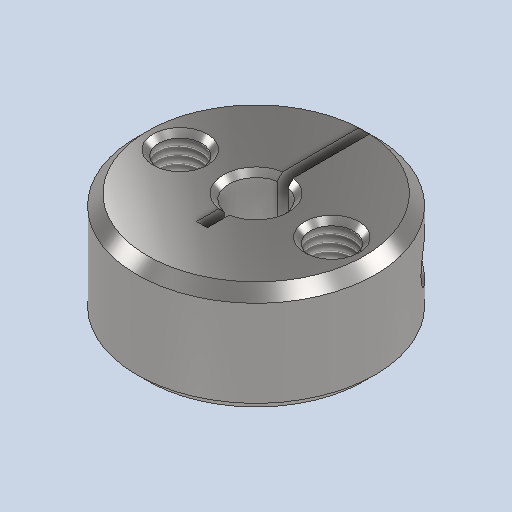
# Autodesk Inventor part: setcorer_5-10-22
Saved by Autodesk Inventor 2025.1 (Build 291241000, 241)
## iProperties
Created: 2023-12-06
Part Number: setcorer_5-10-22
Material: ステンレス鋼 440C
Document SubType Name: Modeling
Designer: fhbdh
Density: 7.75 g/cm^3
Appearance: 半つや出し
Author: fhbdh
Autodesk Inventor part; units mm, degrees
ref_plane "XZ Plane" through (0, 0, 0) normal (0, 1, 0) x (-1, 0, 0)
ref_plane "XY Plane" through (0, 0, 0) normal (0, 0, 1) x (1, 0, 0)
sketch "スケッチ1" plane through (0, 0, 0) normal (0, 1, 0) x (-1, 0, 0)
  circle A0 centre (0, 0) radius 11
  circle A1 centre (0, 0) radius 2.5
  line L0 (0.5, 5) -> (0.5, -10.9886)
  line L1 (0.5, 5) -> (-0.5, 5)
  line L2 (-0.5, 5) -> (-0.5, -10.9886)
  line L3 (0, 0) -> (0, -11) construction
  circle A2 centre (7, 0) radius 2
  line L4 (0, 0) -> (7, 0) construction
  circle A3 centre (-7, 0) radius 2
  point P0 (0.5, 2.4495)
  point P1 (0.5, -2.4495)
  point P2 (-0.5, -2.4495)
  point P3 (-0.5, 2.4495)
  dimension "d0" = 22
  dimension "d1" = 5
  dimension "d2" = 1
  dimension "d3" = 16
  dimension "d4" = 4
  dimension "d7" = 360
  dimension "d9" = 14
  constraints: 10 end point, 4 centre point, 3 point on circle, 2 coincident, 2 horizontal, 2 vertical, 1 parallel, 6 other
  measures "d0" diameter of A0
  measures "d1" diameter of A1
  measures "d2" distance between parallel lines of L2 L0
  measures "d3" distance from line of L3.end L1
  measures "d4" diameter of A2
  measures "d9" distance of A3.centre L4.end
extrude "押し出し1" add sketch "スケッチ1" along normal blind 10 contours A0 L0 A1 L1 L2
ref_plane "作業平面1" through (-11, 0, 0) normal (1, 0, 0) x (0, 1, 0)
sketch "スケッチ2" plane through (-11, 0, 0) normal (1, 0, 0) x (0, 1, 0)
  line L0 (0, 11) -> (10, 11) projected
  line L1 (5, 11) -> (5, -10.9886) construction
  line L2 (0, -10.9886) -> (10, -10.9886) projected
  circle A0 centre (5, -8) radius 4
  point P0 (0, 0)
  dimension "d12" = 8
  dimension "d13" = 8
  constraints: 2 end point, 2 midpoint, 1 centre point, 1 point on line
  measures "d12" diameter of A0
  measures "d13" vertical distance of point (0, 0) A0.centre
extrude "押し出し2" cut sketch "スケッチ2" along normal blind 6
sketch "スケッチ3" plane through (-5, 0, 0) normal (-1, 0, 0) x (0, 0, 1)
  circle A0 centre (-8, 5) radius 2
  line L0 (11, 0) -> (11, 10) projected
  line L1 (11, 5) -> (-10.9886, 5) construction
  line L2 (-10.9886, 0) -> (-10.9886, 10) projected
  point P0 (0, 0)
  point P1 (-9.798, 8.5731)
  point P2 (-9.798, 1.4269)
  point P3 (-10.9886, 5.213)
  point P4 (-10.9886, 4.787)
  dimension "d16" = 4
  dimension "d17" = 8
  constraints: 2 end point, 2 midpoint, 1 centre point, 1 point on line, 1 vertical alignment
  measures "d16" diameter of A0
  measures "d17" horizontal distance of point (0, 0) A0.centre
extrude "押し出し3" cut sketch "スケッチ3" against normal through all
chamfer "面取り1" distance 1 angle 45 2 edges at (0, 10, 11) (0, 0, 11)
chamfer "面取り2" distance 0.5 angle 45 8 edges at (2.5, 10, 0) (-2.5, 10, 0) (-5, 10, 0) (9, 10, 0) (-5, 0, 0) (-2.5, 0, 0) (9, 0, 0) (2.5, 0, 0)
thread "ねじ1" size "M4x0.7" class "6H" standard "ANSI Metric M Profile" length 55
thread "ねじ2" size "M4x0.7" class "6H" standard "ANSI Metric M Profile" length 55
